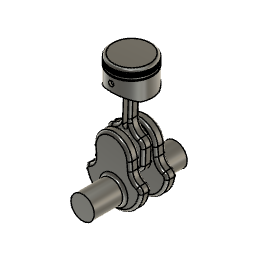
Fusion360 Model (Autodesk Fusion 360 design; units mm, degrees)
Autodesk Fusion 360 part; units mm, degrees
sketch "Sketch1" plane through (0, 0, 0) normal (1, 0, 0) x (0, 1, 0)
  line L0 (0, 0) -> (0, 100)
  line L1 (0, 100) -> (40, 100)
  line L2 (40, 100) -> (40, 93)
  line L3 (40, 93) -> (36, 93)
  line L4 (36, 93) -> (36, 91)
  line L5 (36, 91) -> (40, 91)
  line L6 (40, 91) -> (40, 89)
  line L7 (40, 89) -> (36, 89)
  line L8 (36, 89) -> (36, 87)
  line L9 (36, 87) -> (40, 87)
  line L10 (40, 87) -> (40, 83)
  line L11 (40, 83) -> (36, 83)
  line L12 (36, 83) -> (36, 81)
  line L13 (36, 81) -> (40, 81)
  line L14 (40, 81) -> (40, 45)
  line L15 (40, 45) -> (0, 45)
  dimension "d1" = 40
  dimension "d2" = 7
  dimension "d3" = 4
  dimension "d4" = 2
  dimension "d5" = 4
  dimension "d6" = 4
  dimension "d7" = 4
  dimension "d8" = 4
  dimension "d9" = 4
  dimension "d10" = 2
  dimension "d11" = 2
  dimension "d12" = 4
  dimension "d13" = 2
  dimension "d14" = 36
  dimension "d15" = 100
  constraint coincident L0.start origin
  constraint vertical L0
  constraint perpendicular L0 L1
  constraint perpendicular L1 L2
  constraint perpendicular L2 L3
  constraint perpendicular L3 L4
  constraint perpendicular L4 L5
  constraint perpendicular L5 L6
  constraint perpendicular L6 L7
  constraint perpendicular L7 L8
  constraint perpendicular L8 L9
  constraint perpendicular L9 L10
  constraint perpendicular L10 L11
  constraint perpendicular L11 L12
  constraint perpendicular L12 L13
  constraint perpendicular L13 L14
  constraint coincident L0 L15.end
  constraint perpendicular L0 L15
  measures "d1" distance of L0.end L1.end
  measures "d2" distance of L1.end L2.end
  measures "d3" distance of L2.end L3.end
  measures "d4" distance of L3.end L4.end
  measures "d5" distance of L4.end L5.end
  measures "d6" distance of L6.end L7.end
  measures "d7" distance of L8.end L9.end
  measures "d8" distance of L10.end L11.end
  measures "d9" distance of L12.end L13.end
  measures "d10" distance of L5.end L6.end
  measures "d11" distance of L7.end L8.end
  measures "d12" distance of L9.end L10.end
  measures "d13" distance of L11.end L12.end
  measures "d14" distance of L13.end L14.end
  measures "d15" distance of L0.start L0.end
revolve "Revolve1" add sketch "Sketch1" angle 360 about axis through (0, 0, 0) along (0, 0, 1) makes body 1 in component "Piston"
sketch "Sketch2" plane through (0, 0, 0) normal (0, 1, 0) x (1, 0, 0)
  line L0 (0, 0) -> (0, -130)
  line L1 (40, -45) -> (-40, -45)
  arc A0 (-35.5, -45) -> (35.5, -45) centre (0, 13.0125) ccw
  line L2 (-35.5, -45) -> (-35.5, -20)
  line L3 (-35.5, -20) -> (35.5, -20)
  line L4 (35.5, -20) -> (35.5, -45)
  point P0 (0, -55)
  point P1 (35.5, -45)
  point P2 (-35.5, -45)
  dimension "d17" = 10
  dimension "d18" = 4.5
  constraint coincident L0.start origin
  constraint vertical L0
  constraint coincident L0 P0
  constraint coincident L1 P1
  constraint symmetric L0 P1 P2
  constraint coincident P0 A0
  constraint coincident P1 A0.end
  constraint coincident P2 A0.start
  constraint perpendicular L1 L2
  constraint perpendicular L2 L3
  constraint perpendicular L1 L4
  measures "d17" distance of P0 L1
  measures "d18" distance of L1.start P1
sketch "Sketch3" plane through (0, 0, 45) normal (0, 0, -1) x (1, 0, 0)
  circle A0 centre (0, 0) radius 40
  circle A1 centre (0, 0) radius 35.5
  dimension "d19" = 71
  constraint coincident A0.centre A1.centre
  measures "d19" diameter of A1
extrude "Extrude1" cut sketch "Sketch3" against normal blind 50 contours A1 bodies 1 in component "Piston"
extrude "Extrude2" cut sketch "Sketch2" along normal mid plane 170 bodies 1 in component "Piston"
sketch "Sketch5" plane through (0, 0, 0) normal (0, 1, 0) x (1, 0, 0)
  line L0 (0, 0) -> (0, -105)
  circle A0 centre (0, -69) radius 5
  line L1 (40, -45) -> (35.5, -45)
  dimension "d24" = 10
  dimension "d25" = 24
  constraint coincident L0.start origin
  constraint vertical L0
  constraint coincident L0 A0.centre
  measures "d24" diameter of A0
  measures "d25" distance of A0.centre L1
extrude "Extrude3" cut sketch "Sketch5" along normal mid plane 220 bodies 1 in component "Piston"
fillet "Fillet1" radius 5 1 edges at (-37.2931, 14.4646, 100) on bodies 1 in component "Piston"
sketch "Sketch6" plane through (0, 0, 0) normal (0, 1, 0) x (1, 0, 0)
  spline S0 degree 3 poles (5, -69) (5, -68.3715) (4.8743, -67.7015) (4.3638, -66.4698) (3.9791, -65.908) (3.092, -65.0209) (2.5302, -64.6362) (1.2985, -64.1257) (0.6285, -64) (-0.6285, -64) (-1.2985, -64.1257) (-2.5302, -64.6362) (-3.092, -65.0209) (-3.9791, -65.908) (-4.3638, -66.4698) (-4.8743, -67.7015) (-5, -68.3715) (-5, -69.6285) (-4.8743, -70.2985) (-4.3638, -71.5302) (-3.9791, -72.092) (-3.092, -72.9791) (-2.5302, -73.3638) (-1.2985, -73.8743) (-0.6285, -74) (0.6285, -74) (1.2985, -73.8743) (2.5302, -73.3638) (3.092, -72.9791) (3.9791, -72.092) (4.3638, -71.5302) (4.8743, -70.2985) (5, -69.6285) (5, -69) knots 0 0 0 0 0.188556 0.188556 0.377112 0.377112 0.565667 0.565667 0.754221 0.754221 0.942775 0.942775 1.13133 1.13133 1.319886 1.319886 1.508442 1.508442 1.696998 1.696998 1.885554 1.885554 2.074108 2.074108 2.262663 2.262663 2.451217 2.451217 2.639772 2.639772 2.828328 2.828328 3.016884 3.016884 3.016884 3.016884
  circle A0 centre (0.0087, -69) radius 5
  circle A1 centre (0.0087, -69) radius 8.5
  line L0 (0.0087, -69) -> (0.0087, 54)
  circle A2 centre (0.0087, 54) radius 23
  line L1 (36.0087, 29) -> (36.0087, 54)
  line L2 (0.0087, 54) -> (36.0087, 54)
  line L3 (8.5087, -69) -> (8.5087, 4)
  line L4 (36.0087, 29) -> (33.5087, 29)
  arc A3 (33.5087, 29) -> (8.5087, 4) centre (33.5087, 4) ccw
  line L5 (-35.9913, 29) -> (-33.4913, 29)
  line L6 (-35.9913, 29) -> (-35.9913, 54)
  line L7 (0.0087, 54) -> (-35.9913, 54)
  arc A4 (-8.4913, 4) -> (-33.4913, 29) centre (-33.4913, 4) ccw
  line L8 (-8.4913, -69) -> (-8.4913, 4)
  line L9 (-35.9913, 79) -> (-35.9913, 54)
  line L10 (36.0087, 79) -> (36.0087, 54)
  line L11 (-35.9913, 79) -> (36.0087, 79)
  arc A5 (4.6086, 19) -> (-4.5913, 19) centre (0.0087, 19) ccw
  line L12 (-4.5913, 31.4647) -> (-4.5913, 54)
  line L13 (4.6086, 31.4647) -> (4.6086, 54)
  arc A6 (-4.5913, -54) -> (4.6087, -54) centre (0.0087, -54) ccw
  line L14 (-4.5913, -67.0404) -> (-4.5913, -67.0203)
  line L15 (-4.5913, -54) -> (-4.5913, 19)
  line L16 (4.6086, -67.0608) -> (4.6086, -67.0404)
  line L17 (4.6087, -54) -> (4.6086, 19)
  dimension "d30" = 17
  dimension "d33" = 123
  dimension "d34" = 46
  dimension "d35" = 36
  dimension "d36" = 25
  dimension "d37" = 25
  dimension "d39" = 15
  dimension "d40" = 35
  constraint concentric A0 A1
  constraint coincident A0.centre A1.centre
  constraint vertical L0
  constraint coincident L0.end A2.centre
  constraint vertical L1
  constraint perpendicular L1 L2
  constraint coincident A1 L3.start
  constraint tangent A1 L3
  constraint vertical L3
  constraint perpendicular L3 L4
  constraint tangent L3 A3
  constraint tangent L4 A3
  constraint symmetric L0 L1.start L5.start
  constraint symmetric L0 A2.centre L2.start
  constraint symmetric L0 L1.end L6.end
  constraint symmetric L0 L3.start L8.start
  constraint symmetric L0 L3.end A4.start
  constraint symmetric L0 L4.end L5.end
  constraint symmetric L0 A3 A4
  constraint symmetric L1.start L2 L10.start
  constraint symmetric L2 L1.end L10.end
  constraint symmetric L2 L5.start L9.start
  constraint symmetric L2 L6.end L7.end
  constraint symmetric L0 L13.end L12.end
  constraint coincident L0 A6.centre
  constraint tangent A6 L16
  constraint coincident L0 A5.centre
  constraint tangent A5 L16
  constraint coincident A2 L12.start
  constraint collinear L12 L14
  constraint parallel L0 L16
  constraint coincident A2 L13.start
  constraint collinear L13 L16
  constraint coincident A6.start L14
  constraint coincident A6.end L16
  constraint coincident S0 L14.end
  constraint collinear L14 L15
  constraint coincident A0 L16.end
  constraint collinear L16 L17
  constraint coincident A0 L14.start
  constraint coincident S0 L16.start
  measures "d30" diameter of A1
  measures "d33" distance of A0.centre L0.end
  measures "d34" diameter of A2
  measures "d35" distance of L0 L1
  measures "d36" distance of L1.start L1.end
  measures "d37" radius of A3
  measures "d39" distance of A0.centre A6.centre
  measures "d40" distance of L0.end A5.centre
extrude "Extrude1'" add sketch "Sketch6" along normal mid plane 20 separate body contours A1 L0 A2 L5 L6 L7 A4 L8 A5 A6 L15 | A1 L0 A2 L1 L2 L3 L4 A3 A5 A6 L17 | A2 L2 L7 L9 L10 L11 makes body 2 in component "Connecting Rod"
extrude "Extrude2'" add 1 faces at (12.0087, 3.3333, -79) along direction (0, 0, -1) blind 5 on bodies 2 bodies 2 in component "Connecting Rod"
fillet "Fillet1'" radius 14 4 edges at (-35.9913, 0, -29) (36.0087, 0, -29) (-35.9913, 0, -84) (36.0087, 0, -84) on bodies 2 in component "Connecting Rod"
sketch "Sketch7" plane through (0, 0, 0) normal (0, 1, 0) x (1, 0, 0)
sketch "Sketch8" plane through (0, 0, 0) normal (0, 1, 0) x (1, 0, 0)
  line L0 (55.0087, 18) -> (55.0016, 18)
  line L1 (-54.9913, 18) -> (-54.9984, 18)
  line L2 (-34.9913, 54) -> (-34.9913, 38)
  line L3 (35.0087, 54) -> (35.0087, 38)
  arc A0 (-54.9984, 18) -> (55.0016, 18) centre (0.0016, 18) ccw
  arc A1 (35.0087, 54) -> (-34.9913, 54) centre (0.0087, 54) ccw
  arc A2 (-54.9913, 18) -> (-34.9913, 38) centre (-54.9913, 38) ccw
  arc A3 (35.0087, 38) -> (55.0087, 18) centre (55.0087, 38) ccw
  circle A4 centre (0.0016, -4) radius 22.5
  dimension "d48" = 110
  dimension "d49" = 36
  dimension "d50" = 70
  dimension "d51" = 20
  dimension "d52" = 20
  dimension "d53" = 45
  dimension "d54" = 22
  constraint horizontal L0
  constraint parallel L0 L1
  constraint tangent L2 A1
  constraint perpendicular L1 L2
  constraint tangent L3 A1
  constraint perpendicular L0 L3
  constraint tangent L2 A2
  constraint tangent L1 A2
  constraint tangent L3 A3
  constraint tangent L0 A3
  measures "d48" diameter of A0
  measures "d49" distance of A0.centre A1.centre
  measures "d50" diameter of A1
  measures "d51" radius of A2
  measures "d52" radius of A3
  measures "d53" diameter of A4
  measures "d54" distance of A0.centre A4.centre
extrude "Extrude1''" add sketch "Sketch8" along normal blind 20 from surface at 15 separate body makes body 3 in component "Crankshaft"
extrude "Extrude2''" add 1 faces at (0.5668, 15, -42.1457) along direction (0, -1, 0) blind 20 from surface at 30 on bodies 3 bodies 3 makes body 4 in component "Crankshaft"
sketch "Sketch9" plane through (0, -35, 0) normal (0, -1, 0) x (1, 0, 0)
  circle A0 centre (0.0016, 4) radius 22.5
  arc A1 (-34.9913, -54) -> (35.0087, -54) centre (0.0087, -54) ccw
  line L0 (35.0087, -54) -> (35.0087, -38)
  arc A2 (55.0016, -18) -> (35.0087, -38) centre (55.0087, -38) ccw
  arc A3 (55.0016, -18) -> (-54.9984, -18) centre (0.0016, -18) ccw
  line L1 (-54.9984, -18) -> (-54.9913, -18)
  arc A4 (-34.9913, -38) -> (-54.9913, -18) centre (-54.9913, -38) ccw
  line L2 (-34.9913, -38) -> (-34.9913, -54)
  circle A5 centre (0.0016, 4) radius 22.5
extrude "Extrude3'" add sketch "Sketch9" along normal blind 60 and the other way blind 20 contours A0 A5 bodies 4 in component "Crankshaft"
extrude "Extrude4" add 1 faces at (1.421, -95, -4.4048) along direction (0, -1, 0) blind -180 and the other way blind 110 on bodies 4 bodies 4 3 in component "Crankshaft"
sketch "Sketch10" plane through (0, 0, 0) normal (0, 1, 0) x (1, 0, 0)
  circle A0 centre (0.0087, 54) radius 23
extrude "Extrude5" add sketch "Sketch10" along normal mid plane 60 bodies 3 4 in component "Crankshaft"
fillet "Fillet1''" radius 10 4 edges at (-54.9984, 25, -18) (-54.9984, -25, -18) (55.0016, -25, -18) (55.0016, 25, -18) on bodies 3 in component "Crankshaft"
fillet "Fillet2" radius 5 4 faces at (0.5668, -35, -42.1457) (-29.7244, 15, -12.0315) (-29.7244, -15, -12.0315) (0.5668, 35, -42.1457) on bodies 3 in component "Crankshaft"
fillet "Fillet2'" radius 5 22 edges at (8.5087, -10, 32.5) (13.3928, -10, -18.8443) (33.2735, -10, -32.9531) (36.0087, -10, -55.633) (31.9081, -10, -79.8995) (0.0087, -10, -84) (-31.8908, -10, -79.8995) (-35.9913, -10, -55.633) (-33.2562, -10, -32.9531) (-13.3755, -10, -18.8443) (-8.4913, -10, 32.5) (8.5087, 10, 32.5) (13.3928, 10, -18.8443) (33.2735, 10, -32.9531) (36.0087, 10, -55.633) (31.9081, 10, -79.8995) (0.0087, 10, -84) (-31.8908, 10, -79.8995) (-35.9913, 10, -55.633) (-33.2562, 10, -32.9531) (-13.3755, 10, -18.8443) (-8.4913, 10, 32.5) on bodies 2 in component "Connecting Rod"
sketch "Sketch11" plane through (0, 0, 0) normal (0, 1, 0) x (1, 0, 0)
  spline S0 degree 3 poles (5, -69) (5, -69.6285) (4.8743, -70.2985) (4.3638, -71.5302) (3.9791, -72.092) (3.092, -72.9791) (2.5302, -73.3638) (1.2985, -73.8743) (0.6285, -74) (-0.6285, -74) (-1.2985, -73.8743) (-2.5302, -73.3638) (-3.092, -72.9791) (-3.9791, -72.092) (-4.3638, -71.5302) (-4.8743, -70.2985) (-5, -69.6285) (-5, -68.3715) (-4.8743, -67.7015) (-4.3638, -66.4698) (-3.9791, -65.908) (-3.092, -65.0209) (-2.5302, -64.6362) (-1.2985, -64.1257) (-0.6285, -64) (0.6285, -64) (1.2985, -64.1257) (2.5302, -64.6362) (3.092, -65.0209) (3.9791, -65.908) (4.3638, -66.4698) (4.8743, -67.7015) (5, -68.3715) (5, -69) knots 0 0 0 0 0.188556 0.188556 0.377112 0.377112 0.565667 0.565667 0.754221 0.754221 0.942775 0.942775 1.13133 1.13133 1.319886 1.319886 1.508442 1.508442 1.696998 1.696998 1.885554 1.885554 2.074108 2.074108 2.262663 2.262663 2.451217 2.451217 2.639772 2.639772 2.828328 2.828328 3.016884 3.016884 3.016884 3.016884
extrude "Extrude1'''" add sketch "Sketch11" along normal mid plane 84 separate body makes body 5 in component "Piston pin"
fillet "Fillet1'''" radius 2 2 edges at (-5, -42, 69) (-5, 42, 69) on bodies 5 in component "Piston pin"
sketch "Sketch12" plane through (0, -95, 0) normal (0, -1, 0) x (1, 0, 0)
  circle A0 centre (0.0016, 4) radius 22.5
  circle A1 centre (0.0016, 4) radius 50
  dimension "d81" = 100
  constraint concentric A0 A1
  measures "d81" diameter of A1
extrude "Extrude1''''" add sketch "Sketch12" along normal blind 40 separate body makes body 6 in component "Ground link"
sketch "Sketch13" plane through (0, 0, 100) normal (0, 0, 1) x (-1, 0, 0)
  circle A0 centre (-0.0087, 0.0008) radius 35
  circle A1 centre (-0.0087, 0.0008) radius 75
  dimension "d96" = 150
  constraint concentric A0 A1
  measures "d96" diameter of A1
extrude "Extrude1'''''" add sketch "Sketch13" along normal blind 120 separate body makes body 7 in component "ground Slider "
component "Piston" placed x (1, 0, 0) y (0, 1, 0) z (0, 0, 1) at (0.0087, -0.0008, 60)
component "Connecting Rod" placed x (0.890757, 0, 0.454479) y (0, 1, 0) z (-0.454479, 0, 0.890757) at (31.36, 0, 67.5338)
component "Crankshaft" placed x (-0.266035, 0, 0.963963) y (0, 1, 0) z (-0.963963, 0, -0.266035) at (3.8578, 0, 5.0626)
component "Piston pin" placed x (0.890757, 0, 0.454479) y (0, 1, 0) z (-0.454479, 0, 0.890757) at (26.9139, 0, 65.2653)
component "Ground link" placed x (1, 0, 0) y (0, 1, 0) z (0, 0, 1) at (0, 0, 0)
component "ground Slider " placed x (1, 0, 0) y (0, 1, 0) z (0, 0, 1) at (0, 0, 0)
